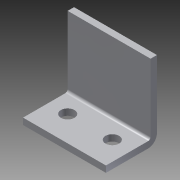
# Autodesk Inventor part: Hard Stop
Saved by Autodesk Inventor 2013 (Build 170138000, 138)
## iProperties
Created: 2013-01-31
Part Number: Hard Stop
Material: Aluminum 6061
Document SubType Name: Sheet Metal
Designer: actoennies
Density: 2.71 g/cm^3
Sheet Metal Rule: Default
Mass: 20.3713 g
Surface Area: 55.0733 cm^2
Volume: 7.51709 cm^3
Author: actoennies
Autodesk Inventor part; units mm, degrees
ref_plane "YZ Plane" through (0, 0, 0) normal (1, 0, 0) x (0, 1, 0)
ref_plane "XZ Plane" through (0, 0, 0) normal (0, 1, 0) x (-1, 0, 0)
ref_plane "XY Plane" through (0, 0, 0) normal (0, 0, 1) x (1, 0, 0)
sketch "Sketch1" plane through (0, 0, 0) normal (0, 1, 0) x (-1, 0, 0)
  line L0 (0, 0) -> (0, 25.4)
  line L1 (0, 25.4) -> (41.275, 25.4)
  line L2 (41.275, 25.4) -> (41.275, 0)
  line L3 (41.275, 0) -> (0, 0)
  circle A0 centre (9.525, 12.7) radius 3.3782
  circle A1 centre (31.75, 12.7) radius 3.3782
  dimension "d0" = 25.4
  dimension "d2" = 6.7564
  dimension "d3" = 6.7564
  dimension "d4" = 22.225
  dimension "d5" = 9.525
  dimension "d6" = 9.525
  dimension "d7" = 12.7
  dimension "d8" = 12.7
  measures "d0" distance of L0.start L0.end
  measures "d2" diameter of A0
  measures "d3" diameter of A1
  measures "d4" distance of A0.centre A1.centre
  measures "d5" distance from line of L0 A0.centre
  measures "d6" distance from line of A1.centre L2
  measures "d7" distance from line of L3 A1.centre
  measures "d8" distance from line of L3 A0.centre
extrude "Plate1" add sketch "Sketch1" along normal blind 3.175
sketch "Sketch2" plane through (-41.275, 0, 3.175) normal (0, 0, -1) x (-1, 0, 0)
  line L0 (-41.275, 0) -> (0, 0)
  line L1 (0, 0) -> (0, 38.1)
  line L2 (0, 38.1) -> (-41.275, 38.1)
  line L3 (-41.275, 38.1) -> (-41.275, 0)
  constraints: 6 end point, 1 horizontal, 1 perpendicular, 1 vertical
edge flange "Flange1" height 38.1 angle 90 thickness 3.175 bend radius 1.27 thickness toward (0, 0, -1) relief straight relief width 3.175 relief depth 1.5875 edges at (-20.6375, 3.175, 0) wall of the first edge with corners at (0, 0, 3.175) (-41.275, 0, 3.175) (-41.275, 38.1, 3.175) (0, 38.1, 3.175)
bend "Bend1"
corner "Corner1"
equation "\"d10\" = BendReliefWidth"
equation "\"d11\" = BendReliefDepth"
equation "\"d12\" = MinimumRemnant"
equation "\"d13\" = BendRadius"
equation "\"d17\" = CornerReliefSize"
equation "\"d18\" = GapSize"
equation "\"d19\" = JacobiRadiusSize"
equation "\"BendRadius\" = Thickness"
equation "\"BendReliefWidth\" = Thickness"
equation "\"BendReliefDepth\" = 0.5 * Thickness"
equation "\"CornerReliefSize\" = 4 * Thickness"
equation "\"MinimumRemnant\" = 2 * Thickness"
equation "\"TransitionRadius\" = BendRadius"
equation "\"JacobiRadiusSize\" = BendRadius"
equation "\"GapSize\" = Thickness"
equation "\"d9\" = BendRadius"
equation "\"Thickness\" = 3.175"
body "Solid1"
